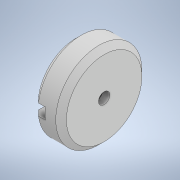
# Autodesk Inventor part: 711133
Saved by Autodesk Inventor 2022 (Build 260153000, 153)
## iProperties
Created: 2021-10-22
Part Number: 711133
Material: Типовые
Document SubType Name: Modeling
Designer: RaNSiD
Density: 1 g/cm^3
Appearance: По умолчанию
Author: RaNSiD
Autodesk Inventor part; units mm, degrees
ref_plane "YZ Plane" through (0, 0, 0) normal (1, 0, 0) x (0, 1, 0)
ref_plane "XZ Plane" through (0, 0, 0) normal (0, 1, 0) x (-1, 0, 0)
ref_plane "XY Plane" through (0, 0, 0) normal (0, 0, 1) x (1, 0, 0)
sketch "Эскиз1" plane through (0, 0, 0) normal (0, 0, 1) x (1, 0, 0)
  line L0 (0, 0) -> (0, 20)
  line L1 (0, 20) -> (2.8284, 22.8284)
  line L2 (0, 0) -> (15, 0)
  line L3 (15, 0) -> (15, 20)
  line L4 (15, 20) -> (12.1716, 22.8284)
  line L5 (12.1716, 22.8284) -> (2.8284, 22.8284)
  dimension "d0" = 20
  dimension "d1" = 4
  dimension "d2" = 135
  dimension "d3" = 15
  dimension "d4" = 4
  dimension "d5" = 135
  constraints: 12 end point, 1 horizontal, 1 parallel, 1 perpendicular, 1 vertical
  measures "d0" distance of L0.start L0.end
  measures "d1" distance of L0.end L1.end
  measures "d2" angle of L0 L1
  measures "d3" distance of L0.start L2.end
  measures "d4" distance of L3.end L4.end
  measures "d5" angle of L4 L3
revolve "Вращение1" add sketch "Эскиз1" angle 360 about axis through (0, 0, 0) along (1, 0, 0)
sketch "Эскиз2" plane through (0, 0, 0) normal (0, 0, 1) x (1, 0, 0)
  line L0 (15, 0) -> (10.5, 0)
  line L1 (15, 3) -> (11.2, 3)
  line L2 (15, 0) -> (15, 3)
  line L3 (11.2, 3.7) -> (10.5, 3.7)
  line L4 (10.5, 3.7) -> (10.5, 0)
  line L5 (10.5, 0) -> (15, 0)
  line L6 (11.2, 3) -> (11.2, 3.7)
  line L7 (15, -20) -> (15, 20) projected
  dimension "d7" = 4.5
  dimension "d9" = 0.7
  dimension "d11" = 3
  dimension "d12" = 0.7
  constraints: 14 end point, 2 horizontal, 2 midpoint, 2 parallel, 1 coincident, 1 perpendicular
  measures "d7" distance between parallel lines of L4 L2
  measures "d9" distance of L3.start L3.end
  measures "d11" distance of L2.start L1.start
  measures "d12" distance of L1.end L3.start
revolve "Вращение2" cut sketch "Эскиз2" angle 360 about axis through (15, 0, 0) along (-1, 0, 0)
sketch "Эскиз3" plane through (0, 0, 0) normal (0, 0, 1) x (1, 0, 0)
  line L0 (0, -20) -> (0, 20) construction
  line L1 (0, -3) -> (6.5, -3)
  line L2 (6.5, -3) -> (6.5, 3)
  line L3 (6.5, 3) -> (0, 3)
  line L4 (0, 3) -> (0, -3)
  point P0 (0, 0)
  point P1 (0, 0)
  point P2 (0, 0)
  dimension "d14" = 6
  dimension "d15" = 6.5
  constraints: 8 end point, 2 midpoint, 2 parallel, 1 coincident, 1 horizontal, 1 perpendicular, 1 point on line
  measures "d14" distance of L1.end L2.end
  measures "d15" distance of L2.end L3.end
extrude "Выдавливание1" cut sketch "Эскиз3" along normal through all both and the other way through all
